Autodesk Fusion 360 part; units mm, degrees
(part 4 of 5)
sketch "SCanner support" plane through (83.6663, 0, 144.9143) normal (0.5, 0, 0.866025) x (0, 1, 0) in component "GM67 + printer"
  line L0 (49, -70.0474) -> (0, -70.0474)
  line L1 (0, -70.0474) -> (0, -120.0474)
  line L2 (0, -120.0474) -> (49, -120.0474)
  line L3 (49, -120.0474) -> (49, -70.0474)
  line L4 (30, -70.0474) -> (30, -120.0474) construction
  line L5 (42.35, -83.2974) -> (17.65, -83.2974) construction
  line L6 (17.65, -83.2974) -> (17.65, -109.6974) construction
  line L7 (17.65, -109.6974) -> (42.35, -109.6974) construction
  line L8 (42.35, -109.6974) -> (42.35, -83.2974) construction
  line L9 (42.35, -83.2974) -> (17.65, -109.6974) construction
  line L10 (17.65, -83.2974) -> (42.35, -109.6974) construction
  circle A0 centre (17.65, -83.2974) radius 1.25
  circle A1 centre (42.35, -83.2974) radius 1.25
  circle A2 centre (42.35, -109.6974) radius 1.25
  circle A3 centre (17.65, -109.6974) radius 1.25
  circle A4 centre (17.65, -83.2974) radius 2.5
  circle A5 centre (42.35, -83.2974) radius 2.5
  circle A6 centre (42.35, -109.6974) radius 2.5
  circle A7 centre (17.65, -109.6974) radius 2.5
  line L11 (0, -70.0474) -> (60, -70.0474)
  circle A8 centre (13.675, -97.0474) radius 2.5
  circle A9 centre (46.325, -97.0474) radius 2.5
  point P0 (30, -70.0474)
  point P1 (30, -96.4974)
  point P2 (13.675, -97.0474)
  point P3 (46.325, -97.0474)
  dimension "d574" = 24.7
  dimension "d575" = 26.4
  dimension "d576" = 2.5
  dimension "d577" = 5
  dimension "d578" = 13.25
  dimension "d655" = 5
  constraint coincident P0 L4.start
  constraint coincident L2 L4.end
  constraint perpendicular L2 L4
  constraint horizontal L5
  constraint perpendicular L5 L6
  constraint parallel L5 L7
  constraint parallel L6 L8
  constraint coincident L9 P1
  constraint coincident L10 P1
  constraint coincident L4 P1
  constraint coincident L5.end L6.start
  constraint coincident L5.start L8.end
  constraint coincident L7.end L8.start
  constraint coincident L6.end L7.start
  constraint equal A0 A1
  constraint equal A1 A2
  constraint equal A2 A3
  constraint concentric A1 A5
  constraint equal A4 A5
  constraint equal A5 A6
  constraint equal A6 A7
  constraint coincident P2 A8.centre
  constraint coincident P3 A9.centre
  constraint equal A8 A9
  measures "d574" distance of L6.end L7.end
  measures "d575" distance of L5.end L6.end
  measures "d576" diameter of A0
  measures "d577" diameter of A4
  measures "d578" distance of L5 L11
  measures "d655" diameter of A9
extrude "Extrude49" cut sketch "SCanner support" against normal up to surface (4 mm away) contours A0 | A1 | A2 | A3 picked at (17.9943, -82.9385) picked at (42.0057, -83.6563) picked at (42.0057, -110.0563) picked at (17.9943, -109.3385) bodies 15 16 5 17 14 in component "GM67 + printer"
extrude "Extrude50" add sketch "SCanner support" along normal blind 3 contours A4 | A5 | A6 | A7 picked at (19.724, -83.4216) picked at (40.4047, -84.0274) picked at (40.4047, -110.4274) picked at (19.724, -109.8216) bodies 17 14 15 5 16 in component "GM67 + printer"
fillet "Fillet11" radius 2 2 edges at (186.6304, 49, 83.1586) (186.6304, 0, 83.1586) on bodies 5 in component "GM67 + printer"
fillet "Fillet12" radius 2 21 edges at (202.8013, 0, 119.1673) (229.4904, 0, 92.6443) (166.4871, 0, 129.0193) (214.8697, 0, 48.0705) (191.0408, 0, 10.4008) (188.2438, 0, 11.6919) (184.4672, 0, 10.6204) (180.543, 0, 8.619) (179.9994, 0, 5.4484) (152.6696, 0, 4) (117.3397, 0, 12) (85.4199, 0, 4) (59.1569, 0, 9.6569) (53.5, 0, 50) (59.1569, 0, 90.3431) (85.4199, 0, 96) (117.3397, 0, 88) (134.8397, 0, 98.5455) (164.8458, 0, 93.4265) (166.8458, 0, 96.8906) (150.8966, 0, 121.2658) on bodies 5 in component "GM67 + printer"
extrude "Extrude51" add sketch "Base" along normal up to surface (150.75 mm away) contours L8 L13 A11 | L13 L43 A39 picked at (4.8547, -10.8354) picked at (4.8547, -89.1646) bodies 5 16 17 in component "GM67 + printer"
fillet "Fillet13" radius 2 8 edges at (27.75, 0, 4) (47.7426, 0, 5.7574) (49.5, 0, 50) (47.7426, 0, 94.2426) (27.75, 0, 96) (4, 0, 50) (9.6569, 0, 9.6569) (9.6569, 0, 90.3431) on bodies 5 in component "GM67 + printer"
fillet "Fillet14" radius 2 1 edges at (143.3292, 49, 108.1586) on bodies 5 in component "GM67 + printer"
sketch "Sketch2 (4)" plane through (0, 0, 0) normal (1, 0, 0) x (0, 1, 0) in component "Powersupply"
  line L0 (25.7117, 31.0761) -> (25.2871, -31.4225)
  line L1 (25.2871, -31.4225) -> (-25.7117, -31.0761)
  line L2 (-25.7117, -31.0761) -> (-25.2871, 31.4225)
  line L3 (-25.2871, 31.4225) -> (25.7117, 31.0761)
  line L4 (25.7117, 31.0761) -> (-25.7117, -31.0761) construction
  line L5 (25.2871, -31.4225) -> (-25.2871, 31.4225) construction
  line L6 (0.0377, -31.251) -> (0.4623, 31.2476) construction
  circle A0 centre (0.3628, 16.5979) radius 1.5
  circle A1 centre (0.0971, -22.5012) radius 1.5
  line L7 (-25.7117, -31.0761) -> (-25.7966, -43.5758)
  line L8 (-25.7966, -43.5758) -> (14.2025, -43.8475)
  line L9 (14.2025, -43.8475) -> (14.2874, -31.3478)
  line L10 (14.2874, -31.3478) -> (-25.7117, -31.0761)
  line L11 (-7.1018, -25.1018) -> (-7.1018, -13.5899) construction
  line L12 (-7.1018, -13.5899) -> (-9.922, -13.5899) construction
  line L13 (-9.922, -13.5899) -> (-9.922, -25.1018) construction
  line L14 (-9.922, -25.1018) -> (-7.1018, -25.1018) construction
  dimension "d595" = 62.5
  dimension "d596" = 51
  dimension "d597" = 25.25
  dimension "d598" = 14.65
  dimension "d599" = 39.1
  dimension "d600" = 3
  dimension "d601" = 12.5
  dimension "d602" = 40
  dimension "d603" = 25.75
  dimension "d604" = 6
  constraint perpendicular L0 L1
  constraint parallel L0 L2
  constraint parallel L1 L3
  constraint coincident L4 origin
  constraint coincident L5 origin
  constraint coincident L1 L6.start
  constraint coincident L3 L6.end
  constraint perpendicular L3 L6
  constraint coincident L6 A0.centre
  constraint coincident L6 A1.centre
  constraint equal A0 A1
  constraint perpendicular L7 L8
  constraint parallel L7 L9
  constraint parallel L8 L10
  constraint perpendicular L1 L7
  measures "d595" distance of L1.end L2.end
  measures "d596" distance of L0.end L1.end
  measures "d597" distance of L0 L6
  measures "d598" distance of L3 A0.centre
  measures "d599" distance of A0.centre A1.centre
  measures "d600" diameter of A1
  measures "d601" distance of L1.end L7.end
  measures "d602" distance of L7.end L8.end
  measures "d603" distance of L2 L6
extrude "Extrude1''''''''" add sketch "Sketch2 (4)" against normal blind 28.5 separate body contours L0 L1 L2 L3 L10 | L1 L7 L8 L9 L10 picked at (-17.3292, 5.4312) picked at (-12.4353, -39.4998) makes body 19 in component "Powersupply"
extrude "Extrude52" cut sketch "Base" against normal blind 1 contours L55 L56 L57 S2 S3 L58 L59 L60 L61 | S4 S5 S6 S7 S8 S9 S10 S11 S12 S13 S14 S15 S16 S17 L62 S18 S19 S20 S21 S22 S23 S24 L63 S25 S26 L64 S27 | L66 L67 L68 S37 S38 S39 S40 S41 L69 L70 L71 S42 S43 S44 S45 S46 L72 L73 | L74 L75 L76 L77 L78 L79 L80 L81 L82 L83 L84 L85 | L86 S47 S48 S49 S50 S51 S52 S53 S54 S55 L87 S56 S57 S58 S59 | L89 L90 L91 S64 S65 S66 S67 S68 S69 S70 L92 L93 L94 S71 S72 S73 S74 S75 L95 L96 L97 S76 S77 S78 S79 S80 L98 L99 | L100 S81 S82 S83 S84 S85 S86 S87 S88 S89 L101 S90 S91 S92 S93 | L103 L104 L105 S98 S99 S100 L106 S101 S102 S103 S104 L107 L108 | L109 S105 S106 S107 S108 L110 L111 L112 L113 L114 L115 L116 L117 L118 L119 L120 S109 S110 S111 S112 | L121 L122 L123 L124 L125 L126 L127 L128 L129 L130 L131 L132 | S113 S114 S115 S116 S117 S118 S119 S120 S121 | L133 L134 L135 S130 S131 S132 S133 S134 S135 S136 L136 L137 L138 S137 S138 S139 S140 S141 L139 L140 L141 S142 S143 S144 S145 S146 L142 L143 | L144 S147 S148 S149 S150 S151 S152 S153 S154 S155 L145 S156 S157 S158 S159 | L147 L148 L149 L150 L151 L152 L153 L154 | L158 S166 S167 S168 S169 S170 L159 L160 L161 S171 S172 S173 S174 S175 S176 L162 L163 L164 L165 | L166 S177 S178 S179 S180 L167 L168 L169 L170 L171 L172 L173 L174 L175 L176 L177 S181 S182 S183 S184 | S185 S186 S187 S188 S189 S190 S191 S192 S193 | L178 L179 L180 S202 S203 S204 S205 S206 S207 S208 L181 L182 L183 S209 S210 S211 S212 S213 L184 L185 L186 S214 S215 S216 S217 S218 L187 L188 | S219 S220 S221 S222 S223 S224 S225 S226 S227 S228 S229 S230 S231 S232 L189 S233 S234 S235 S236 S237 S238 S239 L190 S240 S241 L191 S242 | L193 S252 S253 S254 S255 L194 L195 L196 L197 L198 L199 L200 L201 L202 L203 L204 S256 S257 S258 S259 | L205 L206 L207 L208 | L209 L210 L211 L212 | S260 S261 S262 S263 S264 S265 S266 S267 S268 | L213 L214 L215 S277 S278 S279 S280 S281 L216 L217 L218 S282 S283 S284 S285 S286 L219 L220 picked at (204.0655, -50.3607) picked at (198.4166, -49.6797) picked at (197.0464, -50.5358) picked at (187.6251, -51.1213) picked at (184.3656, -50.4915) picked at (182.292, -50.5028) picked at (174.6623, -50.4915) picked at (172.5955, -50.5085) picked at (169.9477, -50.413) picked at (204.3088, -43.3178) picked at (196.6385, -42.5157) picked at (195.4945, -42.6993) picked at (187.8649, -42.6879) picked at (181.4279, -43.2166) picked at (177.0634, -42.6334) picked at (175.3774, -42.6095) picked at (171.0109, -42.5157) picked at (169.867, -42.6993) picked at (161.5339, -41.8761) picked at (159.8488, -42.6095) picked at (158.015, -45.3948) picked at (158.015, -42.0729) picked at (153.9304, -42.5157) picked at (152.7865, -42.7323) bodies 5 in component "GM67 + printer"
sketch "Sketch1 (7)" plane through (0, 0, 0) normal (1, 0, 0) x (0, 1, 0) in component "display trial"
  line L0 (-8.325, -13) -> (-8.325, -7.5)
  line L1 (13.825, -13) -> (-13.825, -13)
  line L2 (-13.825, 7.5) -> (13.825, -7.5) construction
  line L3 (-13.825, -7.5) -> (13.825, -7.5)
  line L4 (-13.825, -13) -> (-13.825, -7.5)
  line L5 (13.825, -7.5) -> (13.825, 7.5)
  line L6 (-13.825, 16.5) -> (-8.325, 16.5)
  line L7 (13.825, 7.5) -> (-13.825, -7.5) construction
  line L8 (13.825, -7.5) -> (13.825, -13)
  line L9 (-13.825, -7.5) -> (13.825, -7.5)
  line L10 (8.325, -13) -> (8.325, -7.5)
  line L11 (-13.825, 16.5) -> (-13.825, 7.5)
  line L12 (13.825, 7.5) -> (13.825, 16.5)
  line L13 (8.325, 11.8) -> (8.325, 16.5)
  line L14 (-13.825, 7.5) -> (13.825, 7.5)
  line L15 (-8.325, 11.8) -> (-13.825, 11.8)
  line L16 (-8.325, 16.5) -> (-8.325, 11.8)
  line L17 (13.825, 11.8) -> (8.325, 11.8)
  line L18 (13.825, 16.5) -> (-13.825, 16.5)
  line L19 (13.825, 16.5) -> (13.825, 11.8)
  line L20 (-13.825, 11.8) -> (-13.825, 16.5)
  line L21 (13.825, 7.5) -> (-13.825, 7.5)
  line L22 (8.325, 16.5) -> (13.825, 16.5)
  line L23 (-13.825, 7.5) -> (-13.825, -7.5)
  line L24 (23.825, 26.5) -> (-23.825, 26.5)
  line L25 (-23.825, 26.5) -> (-23.825, -23)
  line L26 (-23.825, -23) -> (23.825, -23)
  line L27 (23.825, -23) -> (23.825, 26.5)
  line L28 (-16.325, 7.5) -> (-16.325, -7.5) construction
  line L29 (-16.325, -15.5) -> (-16.325, -7.5) construction
  line L30 (16.325, -15.5) -> (-16.325, -15.5) construction
  line L31 (16.325, -7.5) -> (16.325, -15.5) construction
  line L32 (16.325, -7.5) -> (16.325, 7.5) construction
  line L33 (16.325, 7.5) -> (16.325, 19) construction
  line L34 (16.325, 19) -> (-16.325, 19) construction
  line L35 (-16.325, 19) -> (-16.325, 7.5) construction
  circle A0 centre (-16.325, -15.5) radius 0.95
  circle A1 centre (16.325, -15.5) radius 0.95
  circle A2 centre (16.325, 19) radius 0.95
  circle A3 centre (-16.325, 19) radius 0.95
  dimension "d614" = 27.65
  dimension "d615" = 15
  dimension "d616" = 5.5
  dimension "d617" = 9
  dimension "d618" = 5.5
  dimension "d619" = 5.5
  dimension "d620" = 4.7
  dimension "d621" = 29.5
  dimension "d622" = 24.8
  dimension "d623" = 10
  dimension "d624" = 10
  dimension "d625" = 10
  dimension "d626" = 10
  dimension "d640" = 2.5
  dimension "d641" = 1.9
  constraint perpendicular L21 L23
  constraint parallel L9 L21
  constraint parallel L5 L23
  constraint coincident origin L7
  constraint coincident origin L2
  constraint perpendicular L3 L8
  constraint parallel L1 L3
  constraint parallel L4 L8
  constraint perpendicular L12 L14
  constraint parallel L14 L18
  constraint parallel L11 L12
  constraint coincident L0.start L1
  constraint coincident L0.end L9
  constraint perpendicular L0 L9
  constraint coincident L10.start L1
  constraint coincident L10.end L3
  constraint perpendicular L3 L10
  constraint collinear L0 L16
  constraint coincident L17.start L12
  constraint coincident L13.end L18
  constraint collinear L10 L13
  constraint collinear L15 L17
  constraint horizontal L24
  constraint perpendicular L24 L25
  constraint parallel L24 L26
  constraint parallel L25 L27
  constraint coincident L29.start L30.end
  constraint coincident L30.start L31.end
  constraint coincident L33.end L34.start
  constraint coincident L34.end L35.start
  constraint equal A0 A1
  constraint equal A1 A2
  constraint equal A2 A3
  measures "d614" distance of L2.end L3.start
  measures "d615" distance of L2.start L3.start
  measures "d616" distance of L1.end L3.start
  measures "d617" distance of L2.start L6.start
  measures "d618" distance of L0 L4
  measures "d619" distance of L8 L10
  measures "d620" distance of L6 L15
  measures "d621" distance of L1 L18
  measures "d622" distance of L1 L15
  measures "d623" distance of L5 L27
  measures "d624" distance of L1 L26
  measures "d625" distance of L23 L25
  measures "d626" distance of L18 L24
  measures "d641" diameter of A0
extrude "Extrude1'''''''''" add sketch "Sketch1 (7)" against normal blind 4 separate body contours L24 L25 L26 L27 | A0 | A1 | A2 | A3 picked at (-20.4917, 3.6667) picked at (-16.5962, -15.4559) picked at (16.6171, -15.5472) picked at (16.0634, 19.1784) picked at (-16.4833, 19.2742) makes body 20 in component "display trial"
extrude "Extrude2''''''" add sketch "Sketch1 (7)" against normal blind 0.6 contours L0 L1 L3 L9 L10 | L11 L12 L13 L14 L15 L16 L17 L18 L21 picked at (-2.775, -9.3333) picked at (-2.775, 8.9333) bodies 20 in component "display trial"
extrude "Extrude3''''''" add sketch "Sketch1 (7)" against normal blind 2 contours L0 L1 L3 L4 L9 | L1 L3 L8 L9 L10 | L6 L11 L15 L16 L18 L20 | L12 L13 L17 L18 L19 L22 picked at (-11.9917, -9.3333) picked at (11.9917, -9.3333) picked at (-10.1583, 14.9333) picked at (10.1583, 14.9333) bodies 20 in component "display trial"
sketch "Sketch2 (5)" plane through (-4, 0, 0) normal (-1, 0, 0) x (0, -1, 0) in component "display trial"
  line L0 (13.825, 16.5) -> (13.825, -13)
  line L1 (13.825, -13) -> (-13.825, -13)
  line L2 (-13.825, -13) -> (-13.825, 16.5)
  line L3 (-13.825, 16.5) -> (13.825, 16.5)
  line L4 (-23.825, 26.5) -> (-23.825, -23)
  line L5 (-23.825, -23) -> (23.825, -23)
  line L6 (23.825, -23) -> (23.825, 26.5)
  line L7 (23.825, 26.5) -> (-23.825, 26.5)
  line L8 (-18.825, 21.5) -> (18.825, 21.5)
  line L9 (18.825, 21.5) -> (18.825, -18)
  line L10 (18.825, -18) -> (-18.825, -18)
  line L11 (-18.825, -18) -> (-18.825, 21.5)
  line L12 (18.825, -18) -> (13.825, -13) construction
  line L13 (-13.825, -13) -> (-18.825, -18) construction
  line L14 (18.825, 21.5) -> (13.825, 16.5) construction
  line L15 (13.825, -7.5) -> (8.325, -13)
  line L16 (8.325, -13) -> (-8.325, -13)
  line L17 (-13.825, -7.5) -> (-8.325, -13)
  line L18 (-13.825, 11.8) -> (-13.825, -7.5)
  line L19 (13.825, 11.8) -> (13.825, -7.5)
  line L20 (8.325, 16.5) -> (-8.325, 16.5)
  line L21 (-8.325, 16.5) -> (-13.825, 11.8)
  line L22 (13.825, 11.8) -> (8.325, 16.5)
  circle A0 centre (16.325, -15.5) radius 1.325
  circle A1 centre (-16.325, -15.5) radius 1.325
  circle A2 centre (16.325, 19) radius 1.325
  line L23 (-13.825, 16.5) -> (-18.825, 21.5) construction
  circle A3 centre (-16.325, 19) radius 1.325
  line L24 (6.1811, -14.792) -> (5.8128, -14.8411)
  spline S0 degree 2 poles (5.8128, -14.8411) (5.7493, -14.528) (5.5969, -14.3898) knots 0 0 0 1 1 1
  spline S1 degree 2 poles (5.5969, -14.3898) (5.4444, -14.2517) (5.2254, -14.2517) knots 0 0 0 1 1 1
  spline S2 degree 2 poles (5.2254, -14.2517) (4.9656, -14.2517) (4.7865, -14.4318) knots 0 0 0 1 1 1
  spline S3 degree 2 poles (4.7865, -14.4318) (4.6074, -14.6119) (4.6074, -14.8779) knots 0 0 0 1 1 1
  spline S4 degree 2 poles (4.6074, -14.8779) (4.6074, -15.1317) (4.7732, -15.2964) knots 0 0 0 1 1 1
  spline S5 degree 2 poles (4.7732, -15.2964) (4.9389, -15.4611) (5.1947, -15.4611) knots 0 0 0 1 1 1
  spline S6 degree 2 poles (5.1947, -15.4611) (5.2991, -15.4611) (5.4546, -15.4202) knots 0 0 0 1 1 1
  line L25 (5.4546, -15.4202) -> (5.4137, -15.7435)
  spline S7 degree 2 poles (5.4137, -15.7435) (5.3769, -15.7394) (5.3544, -15.7394) knots 0 0 0 1 1 1
  spline S8 degree 2 poles (5.3544, -15.7394) (5.119, -15.7394) (4.9308, -15.8622) knots 0 0 0 1 1 1
  spline S9 degree 2 poles (4.9308, -15.8622) (4.7425, -15.985) (4.7425, -16.2408) knots 0 0 0 1 1 1
  spline S10 degree 2 poles (4.7425, -16.2408) (4.7425, -16.4434) (4.8796, -16.5764) knots 0 0 0 1 1 1
  spline S11 degree 2 poles (4.8796, -16.5764) (5.0167, -16.7094) (5.2336, -16.7094) knots 0 0 0 1 1 1
  spline S12 degree 2 poles (5.2336, -16.7094) (5.4485, -16.7094) (5.5917, -16.5744) knots 0 0 0 1 1 1
  spline S13 degree 2 poles (5.5917, -16.5744) (5.735, -16.4393) (5.7759, -16.1692) knots 0 0 0 1 1 1
  line L26 (5.7759, -16.1692) -> (6.1443, -16.2347)
  spline S14 degree 2 poles (6.1443, -16.2347) (6.0767, -16.605) (5.8373, -16.8087) knots 0 0 0 1 1 1
  spline S15 degree 2 poles (5.8373, -16.8087) (5.5979, -17.0123) (5.2418, -17.0123) knots 0 0 0 1 1 1
  spline S16 degree 2 poles (5.2418, -17.0123) (4.9962, -17.0123) (4.7896, -16.9069) knots 0 0 0 1 1 1
  spline S17 degree 2 poles (4.7896, -16.9069) (4.5829, -16.8015) (4.4734, -16.6194) knots 0 0 0 1 1 1
  spline S18 degree 2 poles (4.4734, -16.6194) (4.3639, -16.4372) (4.3639, -16.2326) knots 0 0 0 1 1 1
  spline S19 degree 2 poles (4.3639, -16.2326) (4.3639, -16.0382) (4.4683, -15.8786) knots 0 0 0 1 1 1
  spline S20 degree 2 poles (4.4683, -15.8786) (4.5726, -15.719) (4.7773, -15.6248) knots 0 0 0 1 1 1
  spline S21 degree 2 poles (4.7773, -15.6248) (4.5113, -15.5634) (4.3639, -15.3701) knots 0 0 0 1 1 1
  spline S22 degree 2 poles (4.3639, -15.3701) (4.2166, -15.1767) (4.2166, -14.8861) knots 0 0 0 1 1 1
  spline S23 degree 2 poles (4.2166, -14.8861) (4.2166, -14.4932) (4.5031, -14.22) knots 0 0 0 1 1 1
  spline S24 degree 2 poles (4.5031, -14.22) (4.7896, -13.9468) (5.2275, -13.9468) knots 0 0 0 1 1 1
  spline S25 degree 2 poles (5.2275, -13.9468) (5.6224, -13.9468) (5.8834, -14.1821) knots 0 0 0 1 1 1
  spline S26 degree 2 poles (5.8834, -14.1821) (6.1443, -14.4175) (6.1811, -14.792) knots 0 0 0 1 1 1
  line L27 (3.6456, -14) -> (3.6456, -14.4195)
  line L28 (3.6456, -14.4195) -> (3.2261, -14.4195)
  line L29 (3.2261, -14.4195) -> (3.2261, -14)
  line L30 (3.2261, -14) -> (3.6456, -14)
  line L31 (0.7766, -16.2653) -> (1.1429, -16.2367)
  spline S27 degree 2 poles (1.1429, -16.2367) (1.192, -16.4536) (1.2821, -16.5518) knots 0 0 0 1 1 1
  spline S28 degree 2 poles (1.2821, -16.5518) (1.4314, -16.7094) (1.6504, -16.7094) knots 0 0 0 1 1 1
  spline S29 degree 2 poles (1.6504, -16.7094) (1.8264, -16.7094) (1.9594, -16.6112) knots 0 0 0 1 1 1
  spline S30 degree 2 poles (1.9594, -16.6112) (2.1334, -16.4843) (2.2336, -16.2408) knots 0 0 0 1 1 1
  spline S31 degree 2 poles (2.2336, -16.2408) (2.3339, -15.9973) (2.338, -15.5471) knots 0 0 0 1 1 1
  spline S32 degree 2 poles (2.338, -15.5471) (2.205, -15.7497) (2.0126, -15.8479) knots 0 0 0 1 1 1
  spline S33 degree 2 poles (2.0126, -15.8479) (1.8203, -15.9461) (1.6095, -15.9461) knots 0 0 0 1 1 1
  spline S34 degree 2 poles (1.6095, -15.9461) (1.2411, -15.9461) (0.9823, -15.675) knots 0 0 0 1 1 1
  spline S35 degree 2 poles (0.9823, -15.675) (0.7234, -15.4038) (0.7234, -14.9741) knots 0 0 0 1 1 1
  spline S36 degree 2 poles (0.7234, -14.9741) (0.7234, -14.6917) (0.8452, -14.4492) knots 0 0 0 1 1 1
  spline S37 degree 2 poles (0.8452, -14.4492) (0.9669, -14.2067) (1.1797, -14.0778) knots 0 0 0 1 1 1
  spline S38 degree 2 poles (1.1797, -14.0778) (1.3926, -13.9488) (1.6627, -13.9488) knots 0 0 0 1 1 1
  spline S39 degree 2 poles (1.6627, -13.9488) (2.1231, -13.9488) (2.4137, -14.2875) knots 0 0 0 1 1 1
  spline S40 degree 2 poles (2.4137, -14.2875) (2.7043, -14.6262) (2.7043, -15.4038) knots 0 0 0 1 1 1
  spline S41 degree 2 poles (2.7043, -15.4038) (2.7043, -16.2735) (2.383, -16.6685) knots 0 0 0 1 1 1
  spline S42 degree 2 poles (2.383, -16.6685) (2.1027, -17.0123) (1.6279, -17.0123) knots 0 0 0 1 1 1
  spline S43 degree 2 poles (1.6279, -17.0123) (1.2739, -17.0123) (1.0477, -16.8138) knots 0 0 0 1 1 1
  spline S44 degree 2 poles (1.0477, -16.8138) (0.8216, -16.6153) (0.7766, -16.2653) knots 0 0 0 1 1 1
  spline S45 degree 2 poles (2.2807, -14.972) (2.2807, -14.7817) (2.1999, -14.6078) knots 0 0 0 1 1 1
  spline S46 degree 2 poles (2.1999, -14.6078) (2.119, -14.4338) (1.9737, -14.3428) knots 0 0 0 1 1 1
  spline S47 degree 2 poles (1.9737, -14.3428) (1.8284, -14.2517) (1.6688, -14.2517) knots 0 0 0 1 1 1
  spline S48 degree 2 poles (1.6688, -14.2517) (1.4355, -14.2517) (1.2677, -14.44) knots 0 0 0 1 1 1
  spline S49 degree 2 poles (1.2677, -14.44) (1.0999, -14.6282) (1.0999, -14.9516) knots 0 0 0 1 1 1
  spline S50 degree 2 poles (1.0999, -14.9516) (1.0999, -15.2626) (1.2657, -15.4417) knots 0 0 0 1 1 1
  spline S51 degree 2 poles (1.2657, -15.4417) (1.4314, -15.6207) (1.6832, -15.6207) knots 0 0 0 1 1 1
  spline S52 degree 2 poles (1.6832, -15.6207) (1.9328, -15.6207) (2.1068, -15.4417) knots 0 0 0 1 1 1
  spline S53 degree 2 poles (2.1068, -15.4417) (2.2807, -15.2626) (2.2807, -14.972) knots 0 0 0 1 1 1
  line L32 (0.2548, -14) -> (0.2548, -16.1733)
  line L33 (0.2548, -16.1733) -> (-0.0747, -16.1733)
  line L34 (-0.0747, -16.1733) -> (-0.0747, -15.8683)
  spline S54 degree 2 poles (-0.0747, -15.8683) (-0.177, -16.028) (-0.3469, -16.1252) knots 0 0 0 1 1 1
  spline S55 degree 2 poles (-0.3469, -16.1252) (-0.5167, -16.2224) (-0.7336, -16.2224) knots 0 0 0 1 1 1
  spline S56 degree 2 poles (-0.7336, -16.2224) (-0.9751, -16.2224) (-1.1296, -16.1221) knots 0 0 0 1 1 1
  spline S57 degree 2 poles (-1.1296, -16.1221) (-1.2841, -16.0218) (-1.3475, -15.8417) knots 0 0 0 1 1 1
  spline S58 degree 2 poles (-1.3475, -15.8417) (-1.6054, -16.2224) (-2.0188, -16.2224) knots 0 0 0 1 1 1
  spline S59 degree 2 poles (-2.0188, -16.2224) (-2.3421, -16.2224) (-2.516, -16.0433) knots 0 0 0 1 1 1
  spline S60 degree 2 poles (-2.516, -16.0433) (-2.69, -15.8643) (-2.69, -15.4918) knots 0 0 0 1 1 1
  line L35 (-2.69, -15.4918) -> (-2.69, -14)
  line L36 (-2.69, -14) -> (-2.3237, -14)
  line L37 (-2.3237, -14) -> (-2.3237, -15.369)
  spline S61 degree 2 poles (-2.3237, -15.369) (-2.3237, -15.59) (-2.2879, -15.6872) knots 0 0 0 1 1 1
  spline S62 degree 2 poles (-2.2879, -15.6872) (-2.252, -15.7844) (-2.1579, -15.8438) knots 0 0 0 1 1 1
  spline S63 degree 2 poles (-2.1579, -15.8438) (-2.0638, -15.9031) (-1.9369, -15.9031) knots 0 0 0 1 1 1
  spline S64 degree 2 poles (-1.9369, -15.9031) (-1.7077, -15.9031) (-1.5563, -15.7507) knots 0 0 0 1 1 1
  spline S65 degree 2 poles (-1.5563, -15.7507) (-1.4048, -15.5982) (-1.4048, -15.2626) knots 0 0 0 1 1 1
  line L38 (-1.4048, -15.2626) -> (-1.4048, -14)
  line L39 (-1.4048, -14) -> (-1.0365, -14)
  line L40 (-1.0365, -14) -> (-1.0365, -15.412)
  spline S66 degree 2 poles (-1.0365, -15.412) (-1.0365, -15.6576) (-0.9465, -15.7804) knots 0 0 0 1 1 1
  spline S67 degree 2 poles (-0.9465, -15.7804) (-0.8564, -15.9031) (-0.6518, -15.9031) knots 0 0 0 1 1 1
  spline S68 degree 2 poles (-0.6518, -15.9031) (-0.4962, -15.9031) (-0.3643, -15.8213) knots 0 0 0 1 1 1
  spline S69 degree 2 poles (-0.3643, -15.8213) (-0.2323, -15.7394) (-0.1729, -15.5819) knots 0 0 0 1 1 1
  spline S70 degree 2 poles (-0.1729, -15.5819) (-0.1136, -15.4243) (-0.1136, -15.1276) knots 0 0 0 1 1 1
  line L41 (-0.1136, -15.1276) -> (-0.1136, -14)
  line L42 (-0.1136, -14) -> (0.2548, -14)
  line L43 (-3.2364, -14) -> (-3.2364, -16.1733)
  line L44 (-3.2364, -16.1733) -> (-3.5658, -16.1733)
  line L45 (-3.5658, -16.1733) -> (-3.5658, -15.8683)
  spline S71 degree 2 poles (-3.5658, -15.8683) (-3.6681, -16.028) (-3.838, -16.1252) knots 0 0 0 1 1 1
  spline S72 degree 2 poles (-3.838, -16.1252) (-4.0078, -16.2224) (-4.2248, -16.2224) knots 0 0 0 1 1 1
  spline S73 degree 2 poles (-4.2248, -16.2224) (-4.4662, -16.2224) (-4.6207, -16.1221) knots 0 0 0 1 1 1
  spline S74 degree 2 poles (-4.6207, -16.1221) (-4.7752, -16.0218) (-4.8387, -15.8417) knots 0 0 0 1 1 1
  spline S75 degree 2 poles (-4.8387, -15.8417) (-5.0965, -16.2224) (-5.5099, -16.2224) knots 0 0 0 1 1 1
  spline S76 degree 2 poles (-5.5099, -16.2224) (-5.8332, -16.2224) (-6.0072, -16.0433) knots 0 0 0 1 1 1
  spline S77 degree 2 poles (-6.0072, -16.0433) (-6.1811, -15.8643) (-6.1811, -15.4918) knots 0 0 0 1 1 1
  line L46 (-6.1811, -15.4918) -> (-6.1811, -14)
  line L47 (-6.1811, -14) -> (-5.8148, -14)
  line L48 (-5.8148, -14) -> (-5.8148, -15.369)
  spline S78 degree 2 poles (-5.8148, -15.369) (-5.8148, -15.59) (-5.779, -15.6872) knots 0 0 0 1 1 1
  spline S79 degree 2 poles (-5.779, -15.6872) (-5.7432, -15.7844) (-5.649, -15.8438) knots 0 0 0 1 1 1
  spline S80 degree 2 poles (-5.649, -15.8438) (-5.5549, -15.9031) (-5.428, -15.9031) knots 0 0 0 1 1 1
  spline S81 degree 2 poles (-5.428, -15.9031) (-5.1988, -15.9031) (-5.0474, -15.7507) knots 0 0 0 1 1 1
  spline S82 degree 2 poles (-5.0474, -15.7507) (-4.896, -15.5982) (-4.896, -15.2626) knots 0 0 0 1 1 1
  line L49 (-4.896, -15.2626) -> (-4.896, -14)
  line L50 (-4.896, -14) -> (-4.5276, -14)
  line L51 (-4.5276, -14) -> (-4.5276, -15.412)
  spline S83 degree 2 poles (-4.5276, -15.412) (-4.5276, -15.6576) (-4.4376, -15.7804) knots 0 0 0 1 1 1
  spline S84 degree 2 poles (-4.4376, -15.7804) (-4.3475, -15.9031) (-4.1429, -15.9031) knots 0 0 0 1 1 1
  spline S85 degree 2 poles (-4.1429, -15.9031) (-3.9874, -15.9031) (-3.8554, -15.8213) knots 0 0 0 1 1 1
  spline S86 degree 2 poles (-3.8554, -15.8213) (-3.7234, -15.7394) (-3.6641, -15.5819) knots 0 0 0 1 1 1
  spline S87 degree 2 poles (-3.6641, -15.5819) (-3.6047, -15.4243) (-3.6047, -15.1276) knots 0 0 0 1 1 1
  line L52 (-3.6047, -15.1276) -> (-3.6047, -14)
  line L53 (-3.6047, -14) -> (-3.2364, -14)
  line L54 (-84.825, -13) -> (-89.825, -18) construction
  circle A4 centre (-87.325, -15.5) radius 1.325
  line L55 (-57.175, -13) -> (-84.825, -13)
  line L56 (-84.825, 11.8) -> (-84.825, -7.5)
  line L57 (-52.175, 21.5) -> (-52.175, -18)
  line L58 (-57.175, 11.8) -> (-57.175, -7.5)
  line L59 (-84.825, 16.5) -> (-57.175, 16.5)
  line L60 (-84.825, -13) -> (-84.825, 16.5)
  line L61 (-57.175, 16.5) -> (-57.175, -13)
  line L62 (-89.825, -18) -> (-89.825, 21.5)
  line L63 (-84.825, -7.5) -> (-79.325, -13)
  line L64 (-89.825, 21.5) -> (-52.175, 21.5)
  line L65 (-62.675, 16.5) -> (-79.325, 16.5)
  circle A5 centre (-87.325, 19) radius 1.325
  circle A6 centre (-54.675, 19) radius 1.325
  line L66 (-57.175, 11.8) -> (-62.675, 16.5)
  line L67 (-84.825, 16.5) -> (-89.825, 21.5) construction
  circle A7 centre (-54.675, -15.5) radius 1.325
  line L68 (-52.175, 21.5) -> (-57.175, 16.5) construction
  line L69 (-52.175, -18) -> (-89.825, -18)
  line L70 (-62.675, -13) -> (-79.325, -13)
  line L71 (-57.175, -7.5) -> (-62.675, -13)
  line L72 (-79.325, 16.5) -> (-84.825, 11.8)
  line L73 (-52.175, -18) -> (-57.175, -13) construction
  line L74 (-64.8189, -14.792) -> (-65.1872, -14.8411)
  spline S88 degree 2 poles (-65.1872, -14.8411) (-65.2507, -14.528) (-65.4031, -14.3898) knots 0 0 0 1 1 1
  spline S89 degree 2 poles (-65.4031, -14.3898) (-65.5556, -14.2517) (-65.7746, -14.2517) knots 0 0 0 1 1 1
  spline S90 degree 2 poles (-65.7746, -14.2517) (-66.0344, -14.2517) (-66.2135, -14.4318) knots 0 0 0 1 1 1
  spline S91 degree 2 poles (-66.2135, -14.4318) (-66.3926, -14.6119) (-66.3926, -14.8779) knots 0 0 0 1 1 1
  spline S92 degree 2 poles (-66.3926, -14.8779) (-66.3926, -15.1317) (-66.2268, -15.2964) knots 0 0 0 1 1 1
  spline S93 degree 2 poles (-66.2268, -15.2964) (-66.0611, -15.4611) (-65.8053, -15.4611) knots 0 0 0 1 1 1
  spline S94 degree 2 poles (-65.8053, -15.4611) (-65.7009, -15.4611) (-65.5454, -15.4202) knots 0 0 0 1 1 1
  line L75 (-65.5454, -15.4202) -> (-65.5863, -15.7435)
  spline S95 degree 2 poles (-65.5863, -15.7435) (-65.6231, -15.7394) (-65.6456, -15.7394) knots 0 0 0 1 1 1
  spline S96 degree 2 poles (-65.6456, -15.7394) (-65.881, -15.7394) (-66.0692, -15.8622) knots 0 0 0 1 1 1
  spline S97 degree 2 poles (-66.0692, -15.8622) (-66.2575, -15.985) (-66.2575, -16.2408) knots 0 0 0 1 1 1
  spline S98 degree 2 poles (-66.2575, -16.2408) (-66.2575, -16.4434) (-66.1204, -16.5764) knots 0 0 0 1 1 1
  spline S99 degree 2 poles (-66.1204, -16.5764) (-65.9833, -16.7094) (-65.7664, -16.7094) knots 0 0 0 1 1 1
  spline S100 degree 2 poles (-65.7664, -16.7094) (-65.5515, -16.7094) (-65.4083, -16.5744) knots 0 0 0 1 1 1
  spline S101 degree 2 poles (-65.4083, -16.5744) (-65.265, -16.4393) (-65.2241, -16.1692) knots 0 0 0 1 1 1
  line L76 (-65.2241, -16.1692) -> (-64.8557, -16.2347)
  spline S102 degree 2 poles (-64.8557, -16.2347) (-64.9233, -16.605) (-65.1627, -16.8087) knots 0 0 0 1 1 1
  spline S103 degree 2 poles (-65.1627, -16.8087) (-65.4021, -17.0123) (-65.7582, -17.0123) knots 0 0 0 1 1 1
  spline S104 degree 2 poles (-65.7582, -17.0123) (-66.0038, -17.0123) (-66.2104, -16.9069) knots 0 0 0 1 1 1
  spline S105 degree 2 poles (-66.2104, -16.9069) (-66.4171, -16.8015) (-66.5266, -16.6194) knots 0 0 0 1 1 1
  spline S106 degree 2 poles (-66.5266, -16.6194) (-66.6361, -16.4372) (-66.6361, -16.2326) knots 0 0 0 1 1 1
  spline S107 degree 2 poles (-66.6361, -16.2326) (-66.6361, -16.0382) (-66.5317, -15.8786) knots 0 0 0 1 1 1
  spline S108 degree 2 poles (-66.5317, -15.8786) (-66.4274, -15.719) (-66.2227, -15.6248) knots 0 0 0 1 1 1
  spline S109 degree 2 poles (-66.2227, -15.6248) (-66.4887, -15.5634) (-66.6361, -15.3701) knots 0 0 0 1 1 1
  spline S110 degree 2 poles (-66.6361, -15.3701) (-66.7834, -15.1767) (-66.7834, -14.8861) knots 0 0 0 1 1 1
  spline S111 degree 2 poles (-66.7834, -14.8861) (-66.7834, -14.4932) (-66.4969, -14.22) knots 0 0 0 1 1 1
  spline S112 degree 2 poles (-66.4969, -14.22) (-66.2104, -13.9468) (-65.7725, -13.9468) knots 0 0 0 1 1 1
  spline S113 degree 2 poles (-65.7725, -13.9468) (-65.3776, -13.9468) (-65.1166, -14.1821) knots 0 0 0 1 1 1
  spline S114 degree 2 poles (-65.1166, -14.1821) (-64.8557, -14.4175) (-64.8189, -14.792) knots 0 0 0 1 1 1
  line L77 (-67.3544, -14) -> (-67.3544, -14.4195)
  line L78 (-67.3544, -14.4195) -> (-67.7739, -14.4195)
  line L79 (-67.7739, -14.4195) -> (-67.7739, -14)
  line L80 (-67.7739, -14) -> (-67.3544, -14)
  line L81 (-69.4928, -14) -> (-69.4928, -14.7183)
  line L82 (-69.4928, -14.7183) -> (-68.1913, -14.7183)
  line L83 (-68.1913, -14.7183) -> (-68.1913, -15.0559)
  line L84 (-68.1913, -15.0559) -> (-69.5604, -17)
  line L85 (-69.5604, -17) -> (-69.8612, -17)
  line L86 (-69.8612, -17) -> (-69.8612, -15.0559)
  line L87 (-69.8612, -15.0559) -> (-70.2664, -15.0559)
  line L88 (-70.2664, -15.0559) -> (-70.2664, -14.7183)
  line L89 (-70.2664, -14.7183) -> (-69.8612, -14.7183)
  line L90 (-69.8612, -14.7183) -> (-69.8612, -14)
  line L91 (-69.8612, -14) -> (-69.4928, -14)
  line L92 (-69.4928, -15.0559) -> (-69.4928, -16.4086)
  line L93 (-69.4928, -16.4086) -> (-68.5535, -15.0559)
  line L94 (-68.5535, -15.0559) -> (-69.4928, -15.0559)
  line L95 (-70.7452, -14) -> (-70.7452, -16.1733)
  line L96 (-70.7452, -16.1733) -> (-71.0747, -16.1733)
  line L97 (-71.0747, -16.1733) -> (-71.0747, -15.8683)
  spline S115 degree 2 poles (-71.0747, -15.8683) (-71.177, -16.028) (-71.3469, -16.1252) knots 0 0 0 1 1 1
  spline S116 degree 2 poles (-71.3469, -16.1252) (-71.5167, -16.2224) (-71.7336, -16.2224) knots 0 0 0 1 1 1
  spline S117 degree 2 poles (-71.7336, -16.2224) (-71.9751, -16.2224) (-72.1296, -16.1221) knots 0 0 0 1 1 1
  spline S118 degree 2 poles (-72.1296, -16.1221) (-72.2841, -16.0218) (-72.3475, -15.8417) knots 0 0 0 1 1 1
  spline S119 degree 2 poles (-72.3475, -15.8417) (-72.6054, -16.2224) (-73.0188, -16.2224) knots 0 0 0 1 1 1
  spline S120 degree 2 poles (-73.0188, -16.2224) (-73.3421, -16.2224) (-73.516, -16.0433) knots 0 0 0 1 1 1
  spline S121 degree 2 poles (-73.516, -16.0433) (-73.69, -15.8643) (-73.69, -15.4918) knots 0 0 0 1 1 1
  line L98 (-73.69, -15.4918) -> (-73.69, -14)
  line L99 (-73.69, -14) -> (-73.3237, -14)
  line L100 (-73.3237, -14) -> (-73.3237, -15.369)
  spline S122 degree 2 poles (-73.3237, -15.369) (-73.3237, -15.59) (-73.2879, -15.6872) knots 0 0 0 1 1 1
  spline S123 degree 2 poles (-73.2879, -15.6872) (-73.252, -15.7844) (-73.1579, -15.8438) knots 0 0 0 1 1 1
  spline S124 degree 2 poles (-73.1579, -15.8438) (-73.0638, -15.9031) (-72.9369, -15.9031) knots 0 0 0 1 1 1
  spline S125 degree 2 poles (-72.9369, -15.9031) (-72.7077, -15.9031) (-72.5563, -15.7507) knots 0 0 0 1 1 1
  spline S126 degree 2 poles (-72.5563, -15.7507) (-72.4048, -15.5982) (-72.4048, -15.2626) knots 0 0 0 1 1 1
  line L101 (-72.4048, -15.2626) -> (-72.4048, -14)
  line L102 (-72.4048, -14) -> (-72.0365, -14)
  line L103 (-72.0365, -14) -> (-72.0365, -15.412)
  spline S127 degree 2 poles (-72.0365, -15.412) (-72.0365, -15.6576) (-71.9465, -15.7804) knots 0 0 0 1 1 1
  spline S128 degree 2 poles (-71.9465, -15.7804) (-71.8564, -15.9031) (-71.6518, -15.9031) knots 0 0 0 1 1 1
  spline S129 degree 2 poles (-71.6518, -15.9031) (-71.4962, -15.9031) (-71.3643, -15.8213) knots 0 0 0 1 1 1
  spline S130 degree 2 poles (-71.3643, -15.8213) (-71.2323, -15.7394) (-71.1729, -15.5819) knots 0 0 0 1 1 1
  spline S131 degree 2 poles (-71.1729, -15.5819) (-71.1136, -15.4243) (-71.1136, -15.1276) knots 0 0 0 1 1 1
  line L104 (-71.1136, -15.1276) -> (-71.1136, -14)
  line L105 (-71.1136, -14) -> (-70.7452, -14)
  line L106 (-74.2364, -14) -> (-74.2364, -16.1733)
  line L107 (-74.2364, -16.1733) -> (-74.5658, -16.1733)
  line L108 (-74.5658, -16.1733) -> (-74.5658, -15.8683)
  spline S132 degree 2 poles (-74.5658, -15.8683) (-74.6681, -16.028) (-74.838, -16.1252) knots 0 0 0 1 1 1
  spline S133 degree 2 poles (-74.838, -16.1252) (-75.0078, -16.2224) (-75.2248, -16.2224) knots 0 0 0 1 1 1
  spline S134 degree 2 poles (-75.2248, -16.2224) (-75.4662, -16.2224) (-75.6207, -16.1221) knots 0 0 0 1 1 1
  spline S135 degree 2 poles (-75.6207, -16.1221) (-75.7752, -16.0218) (-75.8387, -15.8417) knots 0 0 0 1 1 1
  spline S136 degree 2 poles (-75.8387, -15.8417) (-76.0965, -16.2224) (-76.5099, -16.2224) knots 0 0 0 1 1 1
  spline S137 degree 2 poles (-76.5099, -16.2224) (-76.8332, -16.2224) (-77.0072, -16.0433) knots 0 0 0 1 1 1
  spline S138 degree 2 poles (-77.0072, -16.0433) (-77.1811, -15.8643) (-77.1811, -15.4918) knots 0 0 0 1 1 1
  line L109 (-77.1811, -15.4918) -> (-77.1811, -14)
  line L110 (-77.1811, -14) -> (-76.8148, -14)
  line L111 (-76.8148, -14) -> (-76.8148, -15.369)
  spline S139 degree 2 poles (-76.8148, -15.369) (-76.8148, -15.59) (-76.779, -15.6872) knots 0 0 0 1 1 1
  spline S140 degree 2 poles (-76.779, -15.6872) (-76.7432, -15.7844) (-76.649, -15.8438) knots 0 0 0 1 1 1
  spline S141 degree 2 poles (-76.649, -15.8438) (-76.5549, -15.9031) (-76.428, -15.9031) knots 0 0 0 1 1 1
  spline S142 degree 2 poles (-76.428, -15.9031) (-76.1988, -15.9031) (-76.0474, -15.7507) knots 0 0 0 1 1 1
  spline S143 degree 2 poles (-76.0474, -15.7507) (-75.896, -15.5982) (-75.896, -15.2626) knots 0 0 0 1 1 1
  line L112 (-75.896, -15.2626) -> (-75.896, -14)
  line L113 (-75.896, -14) -> (-75.5276, -14)
  line L114 (-75.5276, -14) -> (-75.5276, -15.412)
  spline S144 degree 2 poles (-75.5276, -15.412) (-75.5276, -15.6576) (-75.4376, -15.7804) knots 0 0 0 1 1 1
  spline S145 degree 2 poles (-75.4376, -15.7804) (-75.3475, -15.9031) (-75.1429, -15.9031) knots 0 0 0 1 1 1
  spline S146 degree 2 poles (-75.1429, -15.9031) (-74.9874, -15.9031) (-74.8554, -15.8213) knots 0 0 0 1 1 1
  spline S147 degree 2 poles (-74.8554, -15.8213) (-74.7234, -15.7394) (-74.6641, -15.5819) knots 0 0 0 1 1 1
  spline S148 degree 2 poles (-74.6641, -15.5819) (-74.6047, -15.4243) (-74.6047, -15.1276) knots 0 0 0 1 1 1
  line L115 (-74.6047, -15.1276) -> (-74.6047, -14)
  line L116 (-74.6047, -14) -> (-74.2364, -14)
  line L117 (-139.825, 11.8) -> (-139.825, -7.5)
  line L118 (-139.825, 16.5) -> (-112.175, 16.5)
  line L119 (-112.175, -7.5) -> (-117.675, -13)
  line L120 (-139.825, -13) -> (-139.825, 16.5)
  line L121 (-107.175, 21.5) -> (-112.175, 16.5) construction
  line L122 (-139.825, -13) -> (-144.825, -18) construction
  line L123 (-144.825, 21.5) -> (-107.175, 21.5)
  line L124 (-107.175, -18) -> (-144.825, -18)
  circle A8 centre (-142.325, 19) radius 1.325
  line L125 (-134.325, 16.5) -> (-139.825, 11.8)
  line L126 (-112.175, -13) -> (-139.825, -13)
  line L127 (-139.825, 16.5) -> (-144.825, 21.5) construction
  circle A9 centre (-109.675, 19) radius 1.325
  line L128 (-117.675, -13) -> (-134.325, -13)
  line L129 (-112.175, 11.8) -> (-112.175, -7.5)
  circle A10 centre (-142.325, -15.5) radius 1.325
  line L130 (-144.825, -18) -> (-144.825, 21.5)
  line L131 (-107.175, 21.5) -> (-107.175, -18)
  circle A11 centre (-109.675, -15.5) radius 1.325
  line L132 (-107.175, -18) -> (-112.175, -13) construction
  line L133 (-117.675, 16.5) -> (-134.325, 16.5)
  line L134 (-139.825, -7.5) -> (-134.325, -13)
  line L135 (-112.175, 11.8) -> (-117.675, 16.5)
  line L136 (-112.175, 16.5) -> (-112.175, -13)
  line L137 (-119.8189, -14.792) -> (-120.1872, -14.8411)
  spline S149 degree 2 poles (-120.1872, -14.8411) (-120.2507, -14.528) (-120.4031, -14.3898) knots 0 0 0 1 1 1
  spline S150 degree 2 poles (-120.4031, -14.3898) (-120.5556, -14.2517) (-120.7746, -14.2517) knots 0 0 0 1 1 1
  spline S151 degree 2 poles (-120.7746, -14.2517) (-121.0344, -14.2517) (-121.2135, -14.4318) knots 0 0 0 1 1 1
  spline S152 degree 2 poles (-121.2135, -14.4318) (-121.3926, -14.6119) (-121.3926, -14.8779) knots 0 0 0 1 1 1
  spline S153 degree 2 poles (-121.3926, -14.8779) (-121.3926, -15.1317) (-121.2268, -15.2964) knots 0 0 0 1 1 1
  spline S154 degree 2 poles (-121.2268, -15.2964) (-121.0611, -15.4611) (-120.8053, -15.4611) knots 0 0 0 1 1 1
  spline S155 degree 2 poles (-120.8053, -15.4611) (-120.7009, -15.4611) (-120.5454, -15.4202) knots 0 0 0 1 1 1
  line L138 (-120.5454, -15.4202) -> (-120.5863, -15.7435)
  spline S156 degree 2 poles (-120.5863, -15.7435) (-120.6231, -15.7394) (-120.6456, -15.7394) knots 0 0 0 1 1 1
  spline S157 degree 2 poles (-120.6456, -15.7394) (-120.881, -15.7394) (-121.0692, -15.8622) knots 0 0 0 1 1 1
  spline S158 degree 2 poles (-121.0692, -15.8622) (-121.2575, -15.985) (-121.2575, -16.2408) knots 0 0 0 1 1 1
  spline S159 degree 2 poles (-121.2575, -16.2408) (-121.2575, -16.4434) (-121.1204, -16.5764) knots 0 0 0 1 1 1
  spline S160 degree 2 poles (-121.1204, -16.5764) (-120.9833, -16.7094) (-120.7664, -16.7094) knots 0 0 0 1 1 1
  spline S161 degree 2 poles (-120.7664, -16.7094) (-120.5515, -16.7094) (-120.4083, -16.5744) knots 0 0 0 1 1 1
  spline S162 degree 2 poles (-120.4083, -16.5744) (-120.265, -16.4393) (-120.2241, -16.1692) knots 0 0 0 1 1 1
  line L139 (-120.2241, -16.1692) -> (-119.8557, -16.2347)
  spline S163 degree 2 poles (-119.8557, -16.2347) (-119.9233, -16.605) (-120.1627, -16.8087) knots 0 0 0 1 1 1
  spline S164 degree 2 poles (-120.1627, -16.8087) (-120.4021, -17.0123) (-120.7582, -17.0123) knots 0 0 0 1 1 1
  spline S165 degree 2 poles (-120.7582, -17.0123) (-121.0038, -17.0123) (-121.2104, -16.9069) knots 0 0 0 1 1 1
  spline S166 degree 2 poles (-121.2104, -16.9069) (-121.4171, -16.8015) (-121.5266, -16.6194) knots 0 0 0 1 1 1
  spline S167 degree 2 poles (-121.5266, -16.6194) (-121.6361, -16.4372) (-121.6361, -16.2326) knots 0 0 0 1 1 1
  spline S168 degree 2 poles (-121.6361, -16.2326) (-121.6361, -16.0382) (-121.5317, -15.8786) knots 0 0 0 1 1 1
  spline S169 degree 2 poles (-121.5317, -15.8786) (-121.4274, -15.719) (-121.2227, -15.6248) knots 0 0 0 1 1 1
  spline S170 degree 2 poles (-121.2227, -15.6248) (-121.4887, -15.5634) (-121.6361, -15.3701) knots 0 0 0 1 1 1
  spline S171 degree 2 poles (-121.6361, -15.3701) (-121.7834, -15.1767) (-121.7834, -14.8861) knots 0 0 0 1 1 1
  spline S172 degree 2 poles (-121.7834, -14.8861) (-121.7834, -14.4932) (-121.4969, -14.22) knots 0 0 0 1 1 1
  spline S173 degree 2 poles (-121.4969, -14.22) (-121.2104, -13.9468) (-120.7725, -13.9468) knots 0 0 0 1 1 1
  spline S174 degree 2 poles (-120.7725, -13.9468) (-120.3776, -13.9468) (-120.1166, -14.1821) knots 0 0 0 1 1 1
  spline S175 degree 2 poles (-120.1166, -14.1821) (-119.8557, -14.4175) (-119.8189, -14.792) knots 0 0 0 1 1 1
  line L140 (-122.3544, -14) -> (-122.3544, -14.4195)
  line L141 (-122.3544, -14.4195) -> (-122.7739, -14.4195)
  line L142 (-122.7739, -14.4195) -> (-122.7739, -14)
  line L143 (-122.7739, -14) -> (-122.3544, -14)
  line L144 (-125.248, -14.354) -> (-125.248, -14)
  line L145 (-125.248, -14) -> (-123.265, -14)
  spline S176 degree 2 poles (-123.265, -14) (-123.2609, -14.133) (-123.308, -14.2558) knots 0 0 0 1 1 1
  spline S177 degree 2 poles (-123.308, -14.2558) (-123.3837, -14.4584) (-123.5505, -14.6548) knots 0 0 0 1 1 1
  spline S178 degree 2 poles (-123.5505, -14.6548) (-123.7173, -14.8513) (-124.0324, -15.1091) knots 0 0 0 1 1 1
  spline S179 degree 2 poles (-124.0324, -15.1091) (-124.5215, -15.5102) (-124.6934, -15.7445) knots 0 0 0 1 1 1
  spline S180 degree 2 poles (-124.6934, -15.7445) (-124.8653, -15.9789) (-124.8653, -16.1876) knots 0 0 0 1 1 1
  spline S181 degree 2 poles (-124.8653, -16.1876) (-124.8653, -16.4065) (-124.7087, -16.557) knots 0 0 0 1 1 1
  spline S182 degree 2 poles (-124.7087, -16.557) (-124.5522, -16.7074) (-124.3005, -16.7074) knots 0 0 0 1 1 1
  spline S183 degree 2 poles (-124.3005, -16.7074) (-124.0344, -16.7074) (-123.8748, -16.5477) knots 0 0 0 1 1 1
  spline S184 degree 2 poles (-123.8748, -16.5477) (-123.7152, -16.3881) (-123.7132, -16.1057) knots 0 0 0 1 1 1
  line L146 (-123.7132, -16.1057) -> (-123.3346, -16.1446)
  spline S185 degree 2 poles (-123.3346, -16.1446) (-123.3735, -16.5682) (-123.6272, -16.7902) knots 0 0 0 1 1 1
  spline S186 degree 2 poles (-123.6272, -16.7902) (-123.881, -17.0123) (-124.3087, -17.0123) knots 0 0 0 1 1 1
  spline S187 degree 2 poles (-124.3087, -17.0123) (-124.7405, -17.0123) (-124.9922, -16.7729) knots 0 0 0 1 1 1
  spline S188 degree 2 poles (-124.9922, -16.7729) (-125.2439, -16.5334) (-125.2439, -16.1794) knots 0 0 0 1 1 1
  spline S189 degree 2 poles (-125.2439, -16.1794) (-125.2439, -15.9993) (-125.1702, -15.8254) knots 0 0 0 1 1 1
  spline S190 degree 2 poles (-125.1702, -15.8254) (-125.0965, -15.6514) (-124.9256, -15.4591) knots 0 0 0 1 1 1
  spline S191 degree 2 poles (-124.9256, -15.4591) (-124.7548, -15.2667) (-124.3578, -14.9311) knots 0 0 0 1 1 1
  spline S192 degree 2 poles (-124.3578, -14.9311) (-124.0263, -14.6528) (-123.9321, -14.5535) knots 0 0 0 1 1 1
  spline S193 degree 2 poles (-123.9321, -14.5535) (-123.838, -14.4543) (-123.7766, -14.354) knots 0 0 0 1 1 1
  line L147 (-123.7766, -14.354) -> (-125.248, -14.354)
  line L148 (-125.7452, -14) -> (-125.7452, -16.1733)
  line L149 (-125.7452, -16.1733) -> (-126.0747, -16.1733)
  line L150 (-126.0747, -16.1733) -> (-126.0747, -15.8683)
  spline S194 degree 2 poles (-126.0747, -15.8683) (-126.177, -16.028) (-126.3469, -16.1252) knots 0 0 0 1 1 1
  spline S195 degree 2 poles (-126.3469, -16.1252) (-126.5167, -16.2224) (-126.7336, -16.2224) knots 0 0 0 1 1 1
  spline S196 degree 2 poles (-126.7336, -16.2224) (-126.9751, -16.2224) (-127.1296, -16.1221) knots 0 0 0 1 1 1
  spline S197 degree 2 poles (-127.1296, -16.1221) (-127.2841, -16.0218) (-127.3475, -15.8417) knots 0 0 0 1 1 1
  spline S198 degree 2 poles (-127.3475, -15.8417) (-127.6054, -16.2224) (-128.0188, -16.2224) knots 0 0 0 1 1 1
  spline S199 degree 2 poles (-128.0188, -16.2224) (-128.3421, -16.2224) (-128.516, -16.0433) knots 0 0 0 1 1 1
  spline S200 degree 2 poles (-128.516, -16.0433) (-128.69, -15.8643) (-128.69, -15.4918) knots 0 0 0 1 1 1
  line L151 (-128.69, -15.4918) -> (-128.69, -14)
  line L152 (-128.69, -14) -> (-128.3237, -14)
  line L153 (-128.3237, -14) -> (-128.3237, -15.369)
  spline S201 degree 2 poles (-128.3237, -15.369) (-128.3237, -15.59) (-128.2879, -15.6872) knots 0 0 0 1 1 1
  spline S202 degree 2 poles (-128.2879, -15.6872) (-128.252, -15.7844) (-128.1579, -15.8438) knots 0 0 0 1 1 1
  spline S203 degree 2 poles (-128.1579, -15.8438) (-128.0638, -15.9031) (-127.9369, -15.9031) knots 0 0 0 1 1 1
  spline S204 degree 2 poles (-127.9369, -15.9031) (-127.7077, -15.9031) (-127.5563, -15.7507) knots 0 0 0 1 1 1
  spline S205 degree 2 poles (-127.5563, -15.7507) (-127.4048, -15.5982) (-127.4048, -15.2626) knots 0 0 0 1 1 1
  line L154 (-127.4048, -15.2626) -> (-127.4048, -14)
  line L155 (-127.4048, -14) -> (-127.0365, -14)
  line L156 (-127.0365, -14) -> (-127.0365, -15.412)
  spline S206 degree 2 poles (-127.0365, -15.412) (-127.0365, -15.6576) (-126.9465, -15.7804) knots 0 0 0 1 1 1
  spline S207 degree 2 poles (-126.9465, -15.7804) (-126.8564, -15.9031) (-126.6518, -15.9031) knots 0 0 0 1 1 1
  spline S208 degree 2 poles (-126.6518, -15.9031) (-126.4962, -15.9031) (-126.3643, -15.8213) knots 0 0 0 1 1 1
  spline S209 degree 2 poles (-126.3643, -15.8213) (-126.2323, -15.7394) (-126.1729, -15.5819) knots 0 0 0 1 1 1
  spline S210 degree 2 poles (-126.1729, -15.5819) (-126.1136, -15.4243) (-126.1136, -15.1276) knots 0 0 0 1 1 1
  line L157 (-126.1136, -15.1276) -> (-126.1136, -14)
  line L158 (-126.1136, -14) -> (-125.7452, -14)
  line L159 (-129.2364, -14) -> (-129.2364, -16.1733)
  line L160 (-129.2364, -16.1733) -> (-129.5658, -16.1733)
  line L161 (-129.5658, -16.1733) -> (-129.5658, -15.8683)
  spline S211 degree 2 poles (-129.5658, -15.8683) (-129.6681, -16.028) (-129.838, -16.1252) knots 0 0 0 1 1 1
  spline S212 degree 2 poles (-129.838, -16.1252) (-130.0078, -16.2224) (-130.2248, -16.2224) knots 0 0 0 1 1 1
  spline S213 degree 2 poles (-130.2248, -16.2224) (-130.4662, -16.2224) (-130.6207, -16.1221) knots 0 0 0 1 1 1
  spline S214 degree 2 poles (-130.6207, -16.1221) (-130.7752, -16.0218) (-130.8387, -15.8417) knots 0 0 0 1 1 1
  spline S215 degree 2 poles (-130.8387, -15.8417) (-131.0965, -16.2224) (-131.5099, -16.2224) knots 0 0 0 1 1 1
  spline S216 degree 2 poles (-131.5099, -16.2224) (-131.8332, -16.2224) (-132.0072, -16.0433) knots 0 0 0 1 1 1
  spline S217 degree 2 poles (-132.0072, -16.0433) (-132.1811, -15.8643) (-132.1811, -15.4918) knots 0 0 0 1 1 1
  line L162 (-132.1811, -15.4918) -> (-132.1811, -14)
  line L163 (-132.1811, -14) -> (-131.8148, -14)
  line L164 (-131.8148, -14) -> (-131.8148, -15.369)
  spline S218 degree 2 poles (-131.8148, -15.369) (-131.8148, -15.59) (-131.779, -15.6872) knots 0 0 0 1 1 1
  spline S219 degree 2 poles (-131.779, -15.6872) (-131.7432, -15.7844) (-131.649, -15.8438) knots 0 0 0 1 1 1
  spline S220 degree 2 poles (-131.649, -15.8438) (-131.5549, -15.9031) (-131.428, -15.9031) knots 0 0 0 1 1 1
  spline S221 degree 2 poles (-131.428, -15.9031) (-131.1988, -15.9031) (-131.0474, -15.7507) knots 0 0 0 1 1 1
  spline S222 degree 2 poles (-131.0474, -15.7507) (-130.896, -15.5982) (-130.896, -15.2626) knots 0 0 0 1 1 1
  line L165 (-130.896, -15.2626) -> (-130.896, -14)
  line L166 (-130.896, -14) -> (-130.5276, -14)
  line L167 (-130.5276, -14) -> (-130.5276, -15.412)
  spline S223 degree 2 poles (-130.5276, -15.412) (-130.5276, -15.6576) (-130.4376, -15.7804) knots 0 0 0 1 1 1
  spline S224 degree 2 poles (-130.4376, -15.7804) (-130.3475, -15.9031) (-130.1429, -15.9031) knots 0 0 0 1 1 1
  spline S225 degree 2 poles (-130.1429, -15.9031) (-129.9874, -15.9031) (-129.8554, -15.8213) knots 0 0 0 1 1 1
  spline S226 degree 2 poles (-129.8554, -15.8213) (-129.7234, -15.7394) (-129.6641, -15.5819) knots 0 0 0 1 1 1
  spline S227 degree 2 poles (-129.6641, -15.5819) (-129.6047, -15.4243) (-129.6047, -15.1276) knots 0 0 0 1 1 1
  line L168 (-129.6047, -15.1276) -> (-129.6047, -14)
  line L169 (-129.6047, -14) -> (-129.2364, -14)
  point P0 (13.825, -13)
  point P1 (-13.825, -13)
  point P2 (-13.825, 16.5)
  point P3 (13.825, 16.5)
  point P4 (8.325, 11.8)
  point P5 (-8.325, 11.8)
  point P6 (-8.325, -7.5)
  point P7 (8.325, -7.5)
  point P8 (-13.825, -7.5)
  point P9 (13.825, -7.5)
  point P10 (8.325, -13)
  point P11 (-8.325, -13)
  point P12 (13.825, 11.8)
  point P13 (8.325, 16.5)
  point P14 (-8.325, 16.5)
  point P15 (-13.825, 11.8)
  point P16 (-71, 0)
  point P17 (-57.175, -13)
  point P18 (-84.825, -13)
  point P19 (-84.825, 16.5)
  point P20 (-62.675, -13)
  point P21 (-62.675, 11.8)
  point P22 (-84.825, -7.5)
  point P23 (-79.325, 16.5)
  point P24 (-57.175, 16.5)
  point P25 (-79.325, 11.8)
  point P26 (-79.325, -7.5)
  point P27 (-62.675, -7.5)
  point P28 (-71, 0)
  point P29 (-57.175, -7.5)
  point P30 (-79.325, -13)
  point P31 (-57.175, 11.8)
  point P32 (-62.675, 16.5)
  point P33 (-84.825, 11.8)
  point P34 (-2.516, -16.0433)
  point P35 (-139.825, -7.5)
  point P36 (-134.325, 16.5)
  point P37 (-112.175, 16.5)
  point P38 (-139.825, -13)
  point P39 (-112.175, -13)
  point P40 (-126, 0)
  point P41 (-139.825, 16.5)
  point P42 (-117.675, -13)
  point P43 (-117.675, 11.8)
  point P44 (-139.825, 11.8)
  point P45 (-134.325, -7.5)
  point P46 (-126, 0)
  point P47 (-112.175, -7.5)
  point P48 (-134.325, -13)
  point P49 (-134.325, 11.8)
  point P50 (-117.675, 16.5)
  point P51 (-117.675, -7.5)
  point P52 (-112.175, 11.8)
  dimension "d633" = 5
  dimension "d634" = 5
  dimension "d635" = 5
  dimension "d636" = 5
  dimension "d637" = 2.65
  dimension "d664" = 5
  dimension "d665" = 5
  dimension "d666" = 5
  dimension "d667" = 5
  dimension "d668" = 2.65
  dimension "d670" = 5
  dimension "d671" = 5
  dimension "d672" = 5
  dimension "d673" = 5
  dimension "d674" = 2.65
  constraint horizontal L8